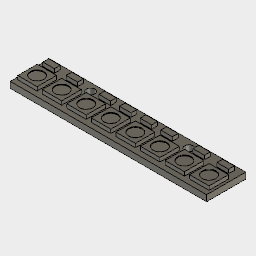
1426 8x NeoPixel Stick (Autodesk Fusion 360 design; units mm, degrees)
Autodesk Fusion 360 part; units mm, degrees
sketch "Sketch1" plane through (0, 0, 0) normal (0, 0, 1) x (1, 0, 0)
  line L0 (0, 0) -> (50.8, 0)
  line L1 (50.8, 0) -> (50.8, 10.16)
  line L2 (50.8, 10.16) -> (0, 10.16)
  line L3 (0, 10.16) -> (0, 0)
  line L4 (25.4, 10.16) -> (25.4, 0) construction
  circle A0 centre (12.7, 8.128) radius 1.1
  circle A1 centre (38.1, 8.128) radius 1.1
  dimension "d1" = 50.8
  dimension "d2" = 10.16
  dimension "d3" = 2.2
  dimension "d4" = 2.2
  dimension "d5" = 12.7
  dimension "d6" = 38.1
  dimension "d7" = 8.128
  dimension "d8" = 8.128
  measures "d1" distance of L1.end L2.end
  measures "d2" distance of L0.start L2.end
  measures "d3" diameter of A0
  measures "d4" diameter of A1
  measures "d5" distance of L3 A0.centre
  measures "d6" distance of L3 A1.centre
  measures "d7" distance of L0 A0.centre
  measures "d8" distance of L0 A1.centre
extrude "Extrude1" add sketch "Sketch1" along normal blind 1.6
sketch "Sketch2" plane through (0, 0, 1.6) normal (0, 0, 1) x (-1, 0, 0)
  circle A0 centre (-12.7, -8.128) radius 1.1
  circle A1 centre (-38.1, -8.128) radius 1.1
  line L0 (0, -10.16) -> (0, 0)
  line L1 (0, 0) -> (-50.8, 0)
  line L2 (-50.8, 0) -> (-50.8, -10.16)
  line L3 (-50.8, -10.16) -> (0, -10.16)
  line L4 (-5.675, -1.31) -> (-0.675, -1.31)
  line L5 (-0.675, -1.31) -> (-0.675, -6.31)
  line L6 (-0.675, -6.31) -> (-5.675, -6.31)
  line L7 (-5.675, -6.31) -> (-5.675, -1.31)
  line L8 (-5.675, -1.31) -> (-0.675, -6.31) construction
  line L9 (-0.675, -1.31) -> (-5.675, -6.31) construction
  circle A2 centre (-3.175, -3.81) radius 1.75
  line L10 (-7.025, -1.31) -> (-7.025, -6.31)
  line L11 (-7.025, -6.31) -> (-12.025, -6.31)
  line L12 (-12.025, -1.31) -> (-7.025, -1.31)
  line L13 (-12.025, -6.31) -> (-12.025, -1.31)
  circle A3 centre (-9.525, -3.81) radius 1.75
  line L14 (-13.375, -1.31) -> (-13.375, -6.31)
  line L15 (-13.375, -6.31) -> (-18.375, -6.31)
  line L16 (-18.375, -1.31) -> (-13.375, -1.31)
  line L17 (-18.375, -6.31) -> (-18.375, -1.31)
  circle A4 centre (-15.875, -3.81) radius 1.75
  line L18 (-19.725, -1.31) -> (-19.725, -6.31)
  line L19 (-19.725, -6.31) -> (-24.725, -6.31)
  line L20 (-24.725, -1.31) -> (-19.725, -1.31)
  line L21 (-24.725, -6.31) -> (-24.725, -1.31)
  circle A5 centre (-22.225, -3.81) radius 1.75
  line L22 (-26.075, -1.31) -> (-26.075, -6.31)
  line L23 (-26.075, -6.31) -> (-31.075, -6.31)
  line L24 (-31.075, -1.31) -> (-26.075, -1.31)
  line L25 (-31.075, -6.31) -> (-31.075, -1.31)
  circle A6 centre (-28.575, -3.81) radius 1.75
  line L26 (-32.425, -1.31) -> (-32.425, -6.31)
  line L27 (-32.425, -6.31) -> (-37.425, -6.31)
  line L28 (-37.425, -1.31) -> (-32.425, -1.31)
  line L29 (-37.425, -6.31) -> (-37.425, -1.31)
  circle A7 centre (-34.925, -3.81) radius 1.75
  line L30 (-38.775, -1.31) -> (-38.775, -6.31)
  line L31 (-38.775, -6.31) -> (-43.775, -6.31)
  line L32 (-43.775, -1.31) -> (-38.775, -1.31)
  line L33 (-43.775, -6.31) -> (-43.775, -1.31)
  circle A8 centre (-41.275, -3.81) radius 1.75
  line L34 (-45.125, -1.31) -> (-45.125, -6.31)
  line L35 (-45.125, -6.31) -> (-50.125, -6.31)
  line L36 (-50.125, -1.31) -> (-45.125, -1.31)
  line L37 (-50.125, -6.31) -> (-50.125, -1.31)
  circle A9 centre (-47.625, -3.81) radius 1.75
  point P0 (-3.175, -3.81)
  dimension "d13" = 5
  dimension "d14" = 5
  dimension "d15" = 3.175
  dimension "d16" = 3.81
  dimension "d17" = 3.5
  dimension "d20" = -6.35
  dimension "d21" = 0
  measures "d13" distance of L5.end L6.end
  measures "d14" distance of L4.end L5.end
  measures "d15" distance of L0 P0
  measures "d16" distance of L1 P0
  measures "d17" diameter of A2
extrude "Extrude2" add sketch "Sketch2" along normal blind 1 draft 1 contours L4 L5 L6 L7 | A2 | L10 L11 L12 L13 | A3 | L14 L15 L16 L17 | A4 | L18 L19 L20 L21 | A5 | L22 L23 L24 L25 | A6 | L26 L27 L28 L29 | A7 | L30 L31 L32 L33 | A8 | L34 L35 L36 L37 | A9
extrude "Extrude3" cut sketch "Sketch2" against normal blind 0.2 from surface at 1 contours A2 | A3 | A4 | A5 | A6 | A7 | A8 | A9
sketch "Sketch3" plane through (0, 0, 1.6) normal (0, 0, 1) x (-1, 0, 0)
  line L0 (-50.125, -6.31) -> (-50.125, -1.31)
  line L1 (-50.125, -1.31) -> (-45.125, -1.31)
  line L2 (-45.125, -1.31) -> (-45.125, -6.31)
  line L3 (-45.125, -6.31) -> (-50.125, -6.31)
  line L4 (-24.725, -6.31) -> (-24.725, -1.31)
  line L5 (-24.725, -1.31) -> (-19.725, -1.31)
  line L6 (-19.725, -1.31) -> (-19.725, -6.31)
  line L7 (-19.725, -6.31) -> (-24.725, -6.31)
  line L8 (-5.675, -6.31) -> (-5.675, -1.31)
  line L9 (-5.675, -1.31) -> (-0.675, -1.31)
  line L10 (-0.675, -1.31) -> (-0.675, -6.31)
  line L11 (-0.675, -6.31) -> (-5.675, -6.31)
  line L12 (-31.075, -6.31) -> (-31.075, -1.31)
  line L13 (-31.075, -1.31) -> (-26.075, -1.31)
  line L14 (-26.075, -1.31) -> (-26.075, -6.31)
  line L15 (-26.075, -6.31) -> (-31.075, -6.31)
  line L16 (-43.775, -6.31) -> (-43.775, -1.31)
  line L17 (-43.775, -1.31) -> (-38.775, -1.31)
  line L18 (-38.775, -1.31) -> (-38.775, -6.31)
  line L19 (-38.775, -6.31) -> (-43.775, -6.31)
  line L20 (-18.375, -6.31) -> (-18.375, -1.31)
  line L21 (-18.375, -1.31) -> (-13.375, -1.31)
  line L22 (-13.375, -1.31) -> (-13.375, -6.31)
  line L23 (-13.375, -6.31) -> (-18.375, -6.31)
  line L24 (-12.025, -6.31) -> (-12.025, -1.31)
  line L25 (-12.025, -1.31) -> (-7.025, -1.31)
  line L26 (-7.025, -1.31) -> (-7.025, -6.31)
  line L27 (-7.025, -6.31) -> (-12.025, -6.31)
  line L28 (-37.425, -6.31) -> (-37.425, -1.31)
  line L29 (-37.425, -1.31) -> (-32.425, -1.31)
  line L30 (-32.425, -1.31) -> (-32.425, -6.31)
  line L31 (-32.425, -6.31) -> (-37.425, -6.31)
  circle A0 centre (-12.7, -8.128) radius 1.1
  circle A1 centre (-38.1, -8.128) radius 1.1
  line L32 (0, -10.16) -> (0, 0)
  line L33 (0, 0) -> (-50.8, 0)
  line L34 (-50.8, 0) -> (-50.8, -10.16)
  line L35 (-50.8, -10.16) -> (0, -10.16)
  line L36 (-0.9, -9.05) -> (-3.9, -9.05)
  line L37 (-3.9, -9.05) -> (-3.9, -7.55)
  line L38 (-3.9, -7.55) -> (-0.9, -7.55)
  line L39 (-0.9, -7.55) -> (-0.9, -9.05)
  line L40 (-2.4, -9.05) -> (-2.4, -7.55) construction
  line L41 (-3.9, -8.3) -> (-0.9, -8.3) construction
  line L42 (-6.9, -7.55) -> (-6.9, -9.05)
  line L43 (-6.9, -9.05) -> (-9.9, -9.05)
  line L44 (-9.9, -7.55) -> (-6.9, -7.55)
  line L45 (-9.9, -9.05) -> (-9.9, -7.55)
  line L46 (-15.4, -9.05) -> (-18.4, -9.05)
  line L47 (-18.4, -9.05) -> (-18.4, -7.55)
  line L48 (-18.4, -7.55) -> (-15.4, -7.55)
  line L49 (-15.4, -7.55) -> (-15.4, -9.05)
  line L50 (-16.9, -9.05) -> (-16.9, -7.55) construction
  line L51 (-18.4, -8.3) -> (-15.4, -8.3) construction
  line L52 (-23.73, -7.55) -> (-20.73, -7.55)
  line L53 (-20.73, -7.55) -> (-20.73, -9.05)
  line L54 (-20.73, -9.05) -> (-23.73, -9.05)
  line L55 (-23.73, -9.05) -> (-23.73, -7.55)
  line L56 (-29.06, -7.55) -> (-26.06, -7.55)
  line L57 (-26.06, -7.55) -> (-26.06, -9.05)
  line L58 (-26.06, -9.05) -> (-29.06, -9.05)
  line L59 (-29.06, -9.05) -> (-29.06, -7.55)
  line L60 (-34.39, -7.55) -> (-31.39, -7.55)
  line L61 (-31.39, -7.55) -> (-31.39, -9.05)
  line L62 (-31.39, -9.05) -> (-34.39, -9.05)
  line L63 (-34.39, -9.05) -> (-34.39, -7.55)
  line L64 (-39.72, -9.05) -> (-42.72, -9.05)
  line L65 (-42.72, -9.05) -> (-42.72, -7.55)
  line L66 (-42.72, -7.55) -> (-39.72, -7.55)
  line L67 (-39.72, -7.55) -> (-39.72, -9.05)
  line L68 (-41.22, -9.05) -> (-41.22, -7.55) construction
  line L69 (-39.72, -8.3) -> (-42.72, -8.3) construction
  line L70 (-32.89, -9.05) -> (-32.89, -7.55) construction
  line L71 (-45.94, -7.55) -> (-45.94, -9.05)
  line L72 (-45.94, -9.05) -> (-48.94, -9.05)
  line L73 (-48.94, -7.55) -> (-45.94, -7.55)
  line L74 (-48.94, -9.05) -> (-48.94, -7.55)
  dimension "d27" = 3
  dimension "d28" = 1.5
  dimension "d29" = 2.4
  dimension "d30" = 8.3
  dimension "d33" = -6
  dimension "d34" = 0
  dimension "d35" = 3
  dimension "d36" = 1.5
  dimension "d37" = 14.5
  dimension "d40" = -5.33
  dimension "d41" = 0
  dimension "d42" = 3
  dimension "d43" = 1.5
  dimension "d44" = 8.33
  dimension "d47" = -6.22
  dimension "d48" = 0
  measures "d27" distance of L36.start L36.end
  measures "d28" distance of L36.start L38.end
  measures "d29" distance of L32 L40
  measures "d30" distance of L33 L41
  measures "d35" distance of L46.start L46.end
  measures "d36" distance of L46.start L48.end
  measures "d37" distance of L40 L50
  measures "d42" distance of L64.start L64.end
  measures "d43" distance of L64.start L66.end
  measures "d44" distance of L68 L70
extrude "Extrude4" add sketch "Sketch3" along normal blind 1 contours L36 L37 L38 L39 | L42 L43 L44 L45 | L46 L47 L48 L49 | L52 L53 L54 L55 | L56 L57 L58 L59 | L60 L61 L62 L63 | L64 L65 L66 L67 | L71 L72 L73 L74
